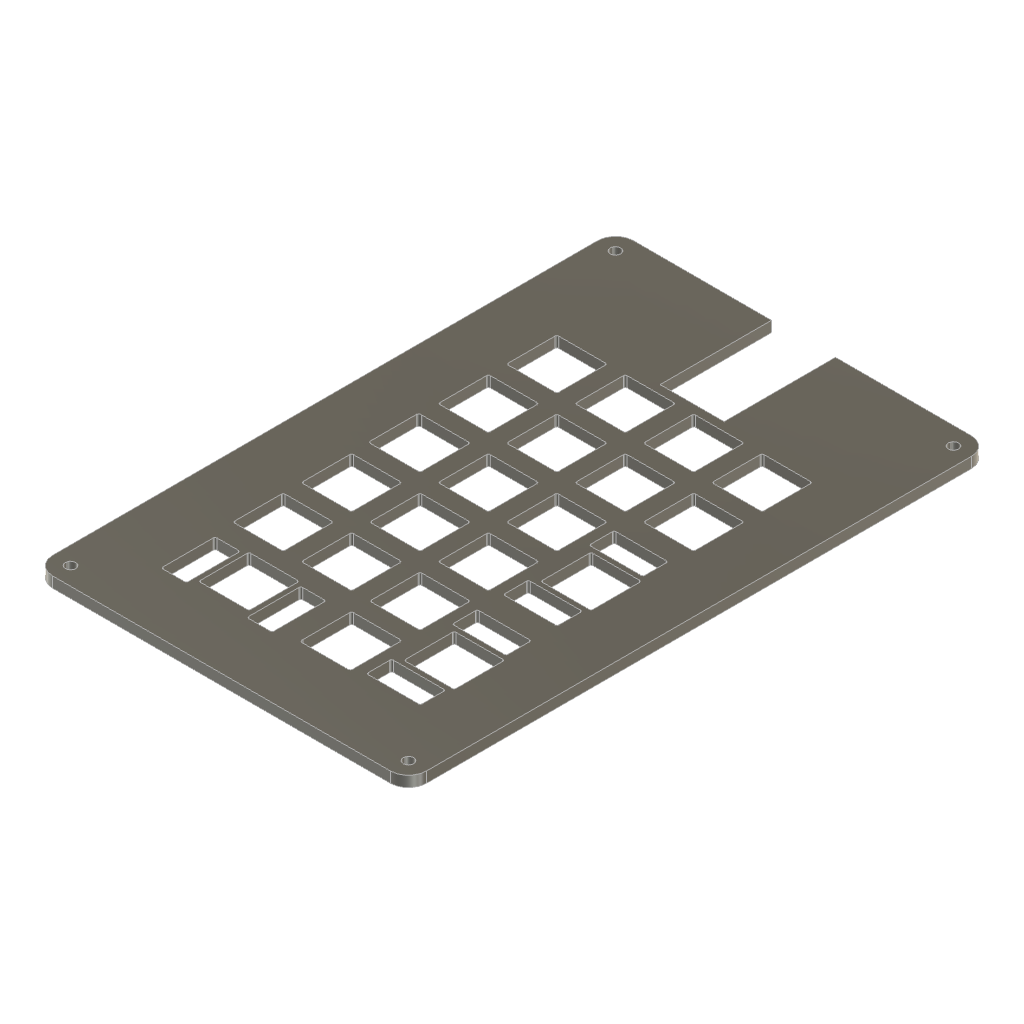
Veekos-full (Autodesk Fusion 360 archive; units mm, degrees)
design "Veekos-top"
part number: 2026-09-16-16-45-23-767
Autodesk Fusion 360 part; units mm, degrees
sketch "Sketch1" plane through (0, 0, 0) normal (0, 0, 1) x (1, 0, 0)
  arc A0 (34.175, -12.588) -> (34.675, -12.088) centre (34.175, -12.088) ccw
  line L0 (16.625, -0.175) -> (16.625, -13.175)
  line L1 (51.502, 90.938) -> (51.502, -70.82)
  line L2 (-2.425, -0.175) -> (-2.425, -13.175)
  line L3 (-35.475, -0.175) -> (-35.475, -13.175)
  line L4 (2.625, -0.175) -> (2.625, -13.175)
  arc A1 (19.675, -12.088) -> (20.175, -12.588) centre (20.175, -12.088) ccw
  arc A2 (34.675, -6.088) -> (34.175, -5.588) centre (34.175, -6.088) ccw
  line L5 (35.175, -4.15) -> (22.175, -4.15)
  arc A3 (35.175, -4.15) -> (35.675, -3.65) centre (35.175, -3.65) ccw
  arc A4 (34.675, -20.312) -> (34.175, -19.812) centre (34.175, -20.312) ccw
  line L6 (34.175, -12.588) -> (20.175, -12.588)
  line L7 (34.175, -5.588) -> (20.175, -5.588)
  line L8 (19.675, -6.088) -> (19.675, -12.088)
  arc A5 (16.125, -13.675) -> (16.625, -13.175) centre (16.125, -13.175) ccw
  arc A6 (20.175, -5.588) -> (19.675, -6.088) centre (20.175, -6.088) ccw
  line L9 (-52.6, -70.82) -> (-52.6, 90.938)
  line L10 (35.675, 9.35) -> (35.675, -3.65)
  arc A7 (21.675, -3.65) -> (22.175, -4.15) centre (22.175, -3.65) ccw
  line L11 (34.175, -19.812) -> (20.175, -19.812)
  line L12 (34.675, -6.088) -> (34.675, -12.088)
  arc A8 (35.175, -42.25) -> (35.675, -41.75) centre (35.175, -41.75) ccw
  arc A9 (35.675, -28.75) -> (35.175, -28.25) centre (35.175, -28.75) ccw
  line L13 (34.175, -50.688) -> (20.175, -50.688)
  line L14 (35.675, -28.75) -> (35.675, -41.75)
  arc A10 (21.675, -41.75) -> (22.175, -42.25) centre (22.175, -41.75) ccw
  line L15 (21.675, -28.75) -> (21.675, -41.75)
  arc A11 (19.675, -26.312) -> (20.175, -26.812) centre (20.175, -26.312) ccw
  line L16 (35.175, -42.25) -> (22.175, -42.25)
  circle A12 centre (46.502, -65.82) radius 1.45
  arc A13 (21.675, 24.925) -> (22.175, 24.425) centre (22.175, 24.925) ccw
  line L17 (3.1315, -52.175) -> (16.0979, -52.175)
  arc A14 (20.175, 18.288) -> (19.675, 17.788) centre (20.175, 17.788) ccw
  line L18 (3.125, -13.675) -> (16.125, -13.675)
  line L19 (-52.6, 90.938) -> (51.502, 90.938)
  line L20 (3.125, 0.325) -> (16.125, 0.325)
  line L21 (51.502, -70.82) -> (-52.6, -70.82)
  line L22 (3.125, -32.725) -> (16.125, -32.725)
  line L23 (3.125, -37.775) -> (16.125, -37.775)
  line L24 (34.675, 17.788) -> (34.675, 11.788)
  line L25 (-9.145, 90.938) -> (8.655, 90.938)
  line L26 (2.625, 18.875) -> (2.625, 5.875)
  arc A15 (19.675, 11.788) -> (20.175, 11.288) centre (20.175, 11.788) ccw
  arc A16 (35.175, 24.425) -> (35.675, 24.925) centre (35.175, 24.925) ccw
  line L27 (3.125, 5.375) -> (16.125, 5.375)
  line L28 (3.125, 19.375) -> (16.125, 19.375)
  arc A17 (22.175, 9.85) -> (21.675, 9.35) centre (22.175, 9.35) ccw
  arc A18 (3.125, 19.375) -> (2.625, 18.875) centre (3.125, 18.875) ccw
  arc A19 (16.125, 24.425) -> (16.625, 24.925) centre (16.125, 24.925) ccw
  line L29 (34.175, 18.288) -> (20.175, 18.288)
  line L30 (8.655, 59.913) -> (-9.145, 59.913)
  line L31 (22.175, 24.425) -> (35.175, 24.425)
  line L32 (3.125, 24.425) -> (16.125, 24.425)
  arc A20 (2.625, 5.875) -> (3.125, 5.375) centre (3.125, 5.875) ccw
  arc A21 (2.625, 24.925) -> (3.125, 24.425) centre (3.125, 24.925) ccw
  line L33 (19.675, 17.788) -> (19.675, 11.788)
  line L34 (35.175, 9.85) -> (22.175, 9.85)
  line L35 (16.625, 18.875) -> (16.625, 5.875)
  arc A22 (16.625, -0.175) -> (16.125, 0.325) centre (16.125, -0.175) ccw
  line L36 (35.675, 37.925) -> (35.675, 24.925)
  arc A23 (34.175, 11.288) -> (34.675, 11.788) centre (34.175, 11.788) ccw
  line L37 (34.175, 11.288) -> (20.175, 11.288)
  line L38 (-16.425, 37.925) -> (-16.425, 24.925)
  arc A24 (34.675, 17.788) -> (34.175, 18.288) centre (34.175, 17.788) ccw
  arc A25 (35.675, 9.35) -> (35.175, 9.85) centre (35.175, 9.35) ccw
  line L39 (-35.475, 37.925) -> (-35.475, 24.925)
  arc A26 (16.125, 5.375) -> (16.625, 5.875) centre (16.125, 5.875) ccw
  arc A27 (16.625, 18.875) -> (16.125, 19.375) centre (16.125, 18.875) ccw
  line L40 (2.625, 37.925) -> (2.625, 24.925)
  line L41 (-21.475, 37.925) -> (-21.475, 24.925)
  line L42 (-2.425, 37.925) -> (-2.425, 24.925)
  line L43 (21.675, 37.925) -> (21.675, 24.925)
  arc A28 (-35.475, 24.925) -> (-34.975, 24.425) centre (-34.975, 24.925) ccw
  line L44 (-34.975, 43.475) -> (-21.975, 43.475)
  line L45 (16.625, 37.925) -> (16.625, 24.925)
  line L46 (21.675, 56.975) -> (21.675, 43.975)
  line L47 (-15.925, 19.375) -> (-2.925, 19.375)
  line L48 (3.125, 38.425) -> (16.125, 38.425)
  line L49 (-34.9851, 5.375) -> (-21.975, 5.375)
  line L50 (8.655, 90.938) -> (8.655, 59.913)
  arc A29 (-10.012, -38.775) -> (-10.512, -39.275) centre (-10.012, -39.275) ccw
  line L51 (-34.388, -39.275) -> (-34.388, -53.275)
  line L52 (-25.95, -38.275) -> (-25.95, -51.275)
  line L53 (-15.925, -32.725) -> (-2.925, -32.725)
  circle A30 centre (-47.6, -65.82) radius 1.45
  arc A31 (2.6077, -51.2737) -> (3.1315, -52.175) centre (3.2951, -51.4771) ccw
  arc A32 (-11.95, -38.275) -> (-12.45, -37.775) centre (-12.45, -38.275) ccw
  arc A33 (2.625, -32.225) -> (3.125, -32.725) centre (3.125, -32.225) ccw
  arc A34 (-16.425, -32.225) -> (-15.925, -32.725) centre (-15.925, -32.225) ccw
  line L54 (-33.888, -38.775) -> (-27.888, -38.775)
  line L55 (-3.512, -39.275) -> (-3.512, -53.275)
  line L56 (-10.012, -38.775) -> (-4.012, -38.775)
  line L57 (-27.388, -39.275) -> (-27.388, -53.275)
  line L58 (-11.95, -38.275) -> (-11.95, -51.275)
  line L59 (-25.45, -37.775) -> (-12.45, -37.775)
  line L60 (-34.975, -32.725) -> (-21.975, -32.725)
  arc A35 (-10.512, -53.275) -> (-10.012, -53.775) centre (-10.012, -53.275) ccw
  line L61 (-33.888, -53.775) -> (-27.888, -53.775)
  line L62 (-21.475, -19.225) -> (-21.475, -32.225)
  line L63 (2.625, -19.225) -> (2.625, -32.225)
  line L64 (-2.425, -19.225) -> (-2.425, -32.225)
  line L65 (-16.425, -19.225) -> (-16.425, -32.225)
  line L66 (-35.475, -19.225) -> (-35.475, -32.225)
  arc A36 (3.125, 0.325) -> (2.625, -0.175) centre (3.125, -0.175) ccw
  line L67 (3.125, -18.725) -> (16.125, -18.725)
  arc A37 (16.625, -19.225) -> (16.125, -18.725) centre (16.125, -19.225) ccw
  line L68 (-21.475, -0.175) -> (-21.475, -13.175)
  line L69 (-16.425, -0.175) -> (-16.425, -13.175)
  arc A38 (20.175, -19.812) -> (19.675, -20.312) centre (20.175, -20.312) ccw
  arc A39 (-21.975, -13.675) -> (-21.475, -13.175) centre (-21.975, -13.175) ccw
  line L70 (-15.925, -13.675) -> (-2.925, -13.675)
  arc A40 (-2.925, -13.675) -> (-2.425, -13.175) centre (-2.925, -13.175) ccw
  arc A41 (3.125, -18.725) -> (2.625, -19.225) centre (3.125, -19.225) ccw
  arc A42 (2.625, -13.175) -> (3.125, -13.675) centre (3.125, -13.175) ccw
  arc A43 (-35.475, -13.175) -> (-34.975, -13.675) centre (-34.975, -13.175) ccw
  line L71 (-34.975, -13.675) -> (-21.975, -13.675)
  arc A44 (-25.95, -51.275) -> (-25.45, -51.775) centre (-25.45, -51.275) ccw
  arc A45 (-12.45, -51.775) -> (-11.95, -51.275) centre (-12.45, -51.275) ccw
  arc A46 (-35.475, -32.225) -> (-34.975, -32.725) centre (-34.975, -32.225) ccw
  arc A47 (-27.888, -53.775) -> (-27.388, -53.275) centre (-27.888, -53.275) ccw
  arc A48 (-27.388, -39.275) -> (-27.888, -38.775) centre (-27.888, -39.275) ccw
  arc A49 (-2.925, -32.725) -> (-2.425, -32.225) centre (-2.925, -32.225) ccw
  arc A50 (-21.975, -32.725) -> (-21.475, -32.225) centre (-21.975, -32.225) ccw
  line L72 (2.625, -38.275) -> (2.6077, -51.2737)
  line L73 (-10.512, -39.275) -> (-10.512, -53.275)
  arc A51 (3.125, -37.775) -> (2.625, -38.275) centre (3.125, -38.275) ccw
  arc A52 (-34.388, -53.275) -> (-33.888, -53.775) centre (-33.888, -53.275) ccw
  arc A53 (-33.888, -38.775) -> (-34.388, -39.275) centre (-33.888, -39.275) ccw
  arc A54 (-25.45, -37.775) -> (-25.95, -38.275) centre (-25.45, -38.275) ccw
  line L74 (-10.012, -53.775) -> (-4.012, -53.775)
  line L75 (-25.45, -51.775) -> (-12.45, -51.775)
  line L76 (21.675, 9.35) -> (21.675, -3.65)
  arc A55 (-4.012, -53.775) -> (-3.512, -53.275) centre (-4.012, -53.275) ccw
  arc A56 (-3.512, -39.275) -> (-4.012, -38.775) centre (-4.012, -39.275) ccw
  arc A57 (20.175, -43.688) -> (19.675, -44.188) centre (20.175, -44.188) ccw
  arc A58 (19.675, -50.188) -> (20.175, -50.688) centre (20.175, -50.188) ccw
  arc A59 (34.175, -26.812) -> (34.675, -26.312) centre (34.175, -26.312) ccw
  line L77 (34.175, -43.688) -> (20.175, -43.688)
  line L78 (19.675, -44.188) -> (19.675, -50.188)
  line L79 (34.175, -26.812) -> (20.175, -26.812)
  line L80 (35.175, -28.25) -> (22.175, -28.25)
  arc A60 (16.625, -38.275) -> (16.125, -37.775) centre (16.125, -38.275) ccw
  line L81 (16.625, -38.275) -> (16.6381, -51.2741)
  arc A61 (16.0979, -52.175) -> (16.6381, -51.2741) centre (15.9585, -51.479) ccw
  arc A62 (34.175, -50.688) -> (34.675, -50.188) centre (34.175, -50.188) ccw
  arc A63 (34.675, -44.188) -> (34.175, -43.688) centre (34.175, -44.188) ccw
  arc A64 (22.175, -28.25) -> (21.675, -28.75) centre (22.175, -28.75) ccw
  arc A65 (16.125, -32.725) -> (16.625, -32.225) centre (16.125, -32.225) ccw
  line L82 (34.675, -44.188) -> (34.675, -50.188)
  line L83 (34.675, -20.312) -> (34.675, -26.312)
  line L84 (19.675, -20.312) -> (19.675, -26.312)
  line L85 (16.625, -19.225) -> (16.625, -32.225)
  arc A66 (-34.975, -18.725) -> (-35.475, -19.225) centre (-34.975, -19.225) ccw
  arc A67 (-16.425, -13.175) -> (-15.925, -13.675) centre (-15.925, -13.175) ccw
  arc A68 (-2.425, -19.225) -> (-2.925, -18.725) centre (-2.925, -19.225) ccw
  line L86 (-15.925, -18.725) -> (-2.925, -18.725)
  line L87 (-34.975, -18.725) -> (-21.975, -18.725)
  arc A69 (-15.925, -18.725) -> (-16.425, -19.225) centre (-15.925, -19.225) ccw
  arc A70 (-21.475, -19.225) -> (-21.975, -18.725) centre (-21.975, -19.225) ccw
  arc A71 (-21.975, 43.475) -> (-21.475, 43.975) centre (-21.975, 43.975) ccw
  arc A72 (-2.925, 5.375) -> (-2.425, 5.875) centre (-2.925, 5.875) ccw
  arc A73 (-21.975, 24.425) -> (-21.475, 24.925) centre (-21.975, 24.925) ccw
  line L88 (-34.9841, 19.375) -> (-21.975, 19.375)
  line L89 (-15.925, 5.375) -> (-2.925, 5.375)
  arc A74 (-16.425, 43.975) -> (-15.925, 43.475) centre (-15.925, 43.975) ccw
  arc A75 (-2.425, 37.925) -> (-2.925, 38.425) centre (-2.925, 37.925) ccw
  circle A76 centre (-47.6, 85.938) radius 1.45
  line L90 (-16.425, 56.975) -> (-16.425, 43.975)
  line L91 (-21.475, 56.975) -> (-21.475, 43.975)
  arc A77 (-2.425, 56.975) -> (-2.925, 57.475) centre (-2.925, 56.975) ccw
  line L92 (-34.975, 38.425) -> (-21.975, 38.425)
  line L93 (-15.925, 38.425) -> (-2.925, 38.425)
  arc A78 (-21.475, 56.975) -> (-21.975, 57.475) centre (-21.975, 56.975) ccw
  arc A79 (-2.925, 43.475) -> (-2.425, 43.975) centre (-2.925, 43.975) ccw
  line L94 (-15.925, 43.475) -> (-2.925, 43.475)
  line L95 (-34.975, 57.475) -> (-21.975, 57.475)
  arc A80 (-21.475, 37.925) -> (-21.975, 38.425) centre (-21.975, 37.925) ccw
  arc A81 (-34.975, 38.425) -> (-35.475, 37.925) centre (-34.975, 37.925) ccw
  arc A82 (-15.925, 0.325) -> (-16.425, -0.175) centre (-15.925, -0.175) ccw
  arc A83 (-2.425, 18.875) -> (-2.925, 19.375) centre (-2.925, 18.875) ccw
  line L96 (-35.875, 18.8763) -> (-35.875, 5.8738)
  arc A84 (-21.975, 5.375) -> (-21.475, 5.875) centre (-21.975, 5.875) ccw
  arc A85 (3.125, 38.425) -> (2.625, 37.925) centre (3.125, 37.925) ccw
  line L97 (-34.975, 0.325) -> (-21.975, 0.325)
  arc A86 (-34.975, 57.475) -> (-35.475, 56.975) centre (-34.975, 56.975) ccw
  arc A87 (35.675, 56.975) -> (35.175, 57.475) centre (35.175, 56.975) ccw
  arc A88 (21.675, 43.975) -> (22.175, 43.475) centre (22.175, 43.975) ccw
  line L98 (35.675, 56.975) -> (35.675, 43.975)
  arc A89 (-15.925, 19.375) -> (-16.425, 18.875) centre (-15.925, 18.875) ccw
  arc A90 (22.175, 38.425) -> (21.675, 37.925) centre (22.175, 37.925) ccw
  line L99 (3.125, 57.475) -> (16.125, 57.475)
  line L100 (-9.145, 59.913) -> (-9.145, 90.938)
  arc A91 (-21.475, -0.175) -> (-21.975, 0.325) centre (-21.975, -0.175) ccw
  arc A92 (35.175, 43.475) -> (35.675, 43.975) centre (35.175, 43.975) ccw
  arc A93 (2.625, 43.975) -> (3.125, 43.475) centre (3.125, 43.975) ccw
  line L101 (22.175, 43.475) -> (35.175, 43.475)
  line L102 (-16.425, 18.875) -> (-16.425, 5.875)
  arc A94 (-15.925, 38.425) -> (-16.425, 37.925) centre (-15.925, 37.925) ccw
  line L103 (-2.425, 56.975) -> (-2.425, 43.975)
  line L104 (-15.925, 0.325) -> (-2.925, 0.325)
  arc A95 (-15.925, 57.475) -> (-16.425, 56.975) centre (-15.925, 56.975) ccw
  arc A96 (-35.475, 43.975) -> (-34.975, 43.475) centre (-34.975, 43.975) ccw
  line L105 (-15.925, 57.475) -> (-2.925, 57.475)
  arc A97 (16.625, 37.925) -> (16.125, 38.425) centre (16.125, 37.925) ccw
  arc A98 (-2.425, -0.175) -> (-2.925, 0.325) centre (-2.925, -0.175) ccw
  arc A99 (3.125, 57.475) -> (2.625, 56.975) centre (3.125, 56.975) ccw
  arc A100 (-16.425, 5.875) -> (-15.925, 5.375) centre (-15.925, 5.875) ccw
  arc A101 (-35.875, 5.8738) -> (-34.9851, 5.375) centre (-35.2073, 6.0218) ccw
  line L106 (3.125, 43.475) -> (16.125, 43.475)
  line L107 (22.175, 38.425) -> (35.175, 38.425)
  arc A102 (-21.475, 18.875) -> (-21.975, 19.375) centre (-21.975, 18.875) ccw
  arc A103 (22.175, 57.475) -> (21.675, 56.975) centre (22.175, 56.975) ccw
  line L108 (16.625, 56.975) -> (16.625, 43.975)
  line L109 (-2.425, 18.875) -> (-2.425, 5.875)
  line L110 (2.625, 56.975) -> (2.625, 43.975)
  circle A104 centre (46.502, 85.938) radius 1.45
  arc A105 (-2.925, 24.425) -> (-2.425, 24.925) centre (-2.925, 24.925) ccw
  line L111 (-35.475, 56.975) -> (-35.475, 43.975)
  line L112 (-34.975, 24.425) -> (-21.975, 24.425)
  arc A106 (16.125, 43.475) -> (16.625, 43.975) centre (16.125, 43.975) ccw
  line L113 (-15.925, 24.425) -> (-2.925, 24.425)
  line L114 (-21.475, 18.875) -> (-21.475, 5.875)
  arc A107 (16.625, 56.975) -> (16.125, 57.475) centre (16.125, 56.975) ccw
  line L115 (22.175, 57.475) -> (35.175, 57.475)
  arc A108 (-16.425, 24.925) -> (-15.925, 24.425) centre (-15.925, 24.925) ccw
  arc A109 (-34.975, 0.325) -> (-35.475, -0.175) centre (-34.975, -0.175) ccw
  arc A110 (-34.9841, 19.375) -> (-35.875, 18.8763) centre (-35.2071, 18.7283) ccw
  arc A111 (35.675, 37.925) -> (35.175, 38.425) centre (35.175, 37.925) ccw
  dimension "d1" = 104.102
  dimension "d2" = 161.758
  dimension "d3" = 16.725
  dimension "d4" = 18.645
  dimension "d5" = 17.8
  dimension "d6" = 31.025
  dimension "d7" = 43.455
  dimension "d8" = 2.9
  dimension "d9" = 5
  dimension "d10" = 5
  dimension "d11" = 2.9
  dimension "d12" = 5
  dimension "d13" = 5
  dimension "d14" = 2.9
  dimension "d15" = 5
  dimension "d16" = 5
  dimension "d17" = 2.9
  dimension "d18" = 5
  dimension "d19" = 5
  constraint horizontal L19
  constraint vertical L1
  constraint horizontal L21
  constraint vertical L9
  constraint horizontal L25
  constraint vertical L50
  constraint horizontal L30
  constraint vertical L100
  constraint coincident L25.start L19
  measures "d1" distance of L1.start L9.end
  measures "d2" distance of L9.end L9.start
  measures "d3" distance of L9 L96
  measures "d4" distance of L17 L21
  measures "d5" distance of L25.end L25.start
  measures "d6" distance of L25.start L30.end
  measures "d7" distance of L9 L100
  measures "d8" diameter of A76
  measures "d9" distance of A76.centre L19
  measures "d10" distance of A76.centre L9
  measures "d11" diameter of A30
  measures "d12" distance of A30.centre L21
  measures "d13" distance of A30.centre L9
  measures "d14" diameter of A12
  measures "d15" distance of A12.centre L21
  measures "d16" distance of A12.centre L1
  measures "d17" diameter of A104
  measures "d18" distance of A104.centre L1
  measures "d19" distance of A104.centre L19
extrude "Extrude1" add sketch "Sketch1" along normal blind 3 contours L1 L9 L19 L21 L30 L50 L100
fillet "Fillet1" radius 5 4 edges at (51.502, -70.82, 1.5) (-52.6, -70.82, 1.5) (51.502, 90.938, 1.5) (-52.6, 90.938, 1.5)

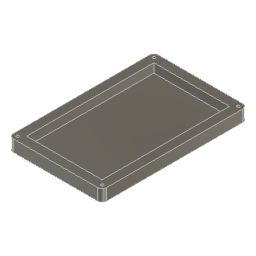
design "Veekos-bottom"
part number: 2026-09-15-13-32-07-212
Autodesk Fusion 360 part; units mm, degrees
sketch "Sketch1" plane through (0, 0, 0) normal (0, 0, 1) x (1, 0, 0)
  line L0 (-51.3011, 107.6317) -> (32.8009, 107.6317)
  line L1 (32.8009, 107.6317) -> (32.8009, -34.1263)
  line L2 (32.8009, -34.1263) -> (-51.3011, -34.1263)
  line L3 (-51.3011, -34.1263) -> (-51.3011, 107.6317)
  line L4 (-61.3011, 117.6317) -> (42.8009, 117.6317)
  line L5 (42.8009, 117.6317) -> (42.8009, -44.1263)
  line L6 (42.8009, -44.1263) -> (-61.3011, -44.1263)
  line L7 (-61.3011, -44.1263) -> (-61.3011, 117.6317)
  circle A0 centre (37.8009, 112.6317) radius 1.45
  circle A1 centre (37.8009, -39.1263) radius 1.45
  circle A2 centre (-56.3011, -39.1263) radius 1.45
  circle A3 centre (-56.3011, 112.6317) radius 1.45
  dimension "d1" = 84.102
  dimension "d2" = 141.758
  dimension "d3" = 104.102
  dimension "d4" = 161.758
  dimension "d5" = 10
  dimension "d6" = 10
  dimension "d7" = 2.9
  dimension "d8" = 5
  dimension "d9" = 5
  dimension "d10" = 2.9
  dimension "d11" = 5
  dimension "d12" = 5
  dimension "d13" = 2.9
  dimension "d14" = 5
  dimension "d15" = 5
  dimension "d16" = 2.9
  dimension "d17" = 5
  dimension "d18" = 5
  constraint horizontal L0
  constraint vertical L1
  constraint horizontal L2
  constraint vertical L3
  constraint horizontal L4
  constraint vertical L5
  constraint horizontal L6
  constraint vertical L7
  measures "d1" distance of L0.start L0.end
  measures "d2" distance of L0.start L2.end
  measures "d3" distance of L4.start L4.end
  measures "d4" distance of L4.start L6.end
  measures "d5" distance of L0 L4
  measures "d6" distance of L3 L7
  measures "d7" diameter of A0
  measures "d8" distance of L5 A0.centre
  measures "d9" distance of L4 A0.centre
  measures "d10" diameter of A1
  measures "d11" distance of L6 A1.centre
  measures "d12" distance of L5 A1.centre
  measures "d13" diameter of A2
  measures "d14" distance of L7 A2.centre
  measures "d15" distance of L6 A2.centre
  measures "d16" diameter of A3
  measures "d17" distance of L4 A3.centre
  measures "d18" distance of L7 A3.centre
extrude "Extrude1" add sketch "Sketch1" along normal blind 3 contours L0 L1 L2 L3
extrude "Extrude2" add sketch "Sketch1" along normal blind 13
fillet "Fillet1" radius 5 4 edges at (42.8009, -44.1263, 6.5) (42.8009, 117.6317, 6.5) (-61.3011, 117.6317, 6.5) (-61.3011, -44.1263, 6.5)
